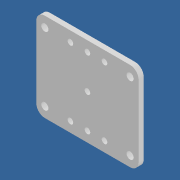
# Autodesk Inventor part: Diode_laser_Mount
Saved by Autodesk Inventor 2020 (Build 240168000, 168)
## iProperties
Created: 2021-07-14
Part Number: Diode_laser_Mount
Material: 一般
Document SubType Name: Modeling
Designer: ken113
Density: 1 g/cm^3
Appearance: 既定
Author: ken113
Autodesk Inventor part; units mm, degrees
ref_plane "YZ Plane" through (0, 0, 0) normal (1, 0, 0) x (0, 1, 0)
ref_plane "XZ Plane" through (0, 0, 0) normal (0, 1, 0) x (-1, 0, 0)
ref_plane "XY Plane" through (0, 0, 0) normal (0, 0, 1) x (1, 0, 0)
sketch "スケッチ1" plane through (0, 0, 0) normal (0, 0, 1) x (1, 0, 0)
  line L0 (30, -26) -> (-30, -26)
  line L1 (-30, -26) -> (-30, 26)
  line L2 (-30, 26) -> (30, 26)
  line L3 (30, 26) -> (30, -26)
  line L4 (30, -26) -> (-30, 26) construction
  line L5 (-30, -26) -> (30, 26) construction
  point P0 (0, 0)
  dimension "d0" = 60
  dimension "d1" = 52
  constraints: 12 end point, 2 midpoint, 2 parallel, 1 horizontal, 1 perpendicular
  measures "d0" distance of L1.end L2.end
  measures "d1" distance of L0.end L1.end
extrude "押し出し1" add sketch "スケッチ1" along normal blind 3
sketch "スケッチ2" plane through (0, 0, 3) normal (0, 0, 1) x (1, 0, 0)
  line L0 (-10, -20) -> (10, -20)
  line L1 (10, -20) -> (10, 20)
  line L2 (10, 20) -> (-10, 20)
  line L3 (-10, 20) -> (-10, -20)
  line L4 (-10, -20) -> (10, 20) construction
  line L5 (10, -20) -> (-10, 20) construction
  line L6 (-30, -26) -> (30, -26) projected
  point P0 (0, 0)
  point P1 (0, 20)
  point P2 (0, -20)
  dimension "d4" = 20
  dimension "d5" = 40
  dimension "d6" = 6
  constraints: 12 end point, 3 midpoint, 2 parallel, 1 horizontal, 1 perpendicular
  measures "d4" distance of L2.end L1.end
  measures "d5" distance of L1.end L0.end
  measures "d6" distance between parallel lines of L0 L6
hole "穴1" at (-10, 20, 3) at (-10, -20, 3) at (10, -20, 3) at (10, 20, 3) at (0, -20, 3) at (0, 0, 3) at (0, 20, 3) direction (0, 0, -1) diameter 3.3 depth 8.8
sketch "スケッチ4" plane through (0, 0, 3) normal (0, 0, 1) x (1, 0, 0)
  line L0 (-25, -20) -> (25, -20)
  line L1 (25, -20) -> (25, 20)
  line L2 (25, 20) -> (-25, 20)
  line L3 (-25, 20) -> (-25, -20)
  line L4 (-25, -20) -> (25, 20) construction
  line L5 (25, -20) -> (-25, 20) construction
  point P0 (0, 0)
  point P1 (0, 20)
  point P2 (0, -20)
  point P3 (0, 0)
  dimension "d14" = 50
  dimension "d15" = 40
  constraints: 12 end point, 4 midpoint, 2 parallel, 1 coincident, 1 horizontal, 1 perpendicular
  measures "d14" distance of L2.end L1.end
  measures "d15" distance of L1.end L0.end
hole "穴2" at (-25, 20, 3) at (-25, -20, 3) at (25, -20, 3) at (25, 20, 3) direction (0, 0, -1) diameter 4.2 depth 8.8
fillet "フィレット1" radius 5 4 edges at (-30, 26, 1.5) (-30, -26, 1.5) (30, -26, 1.5) (30, 26, 1.5)
